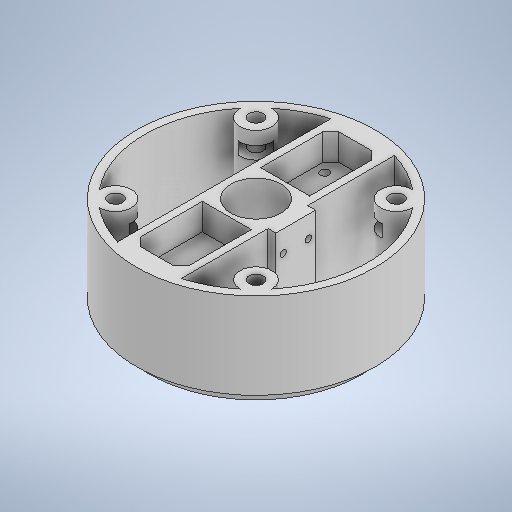
# Autodesk Inventor part: SCARA swivel top
Saved by Autodesk Inventor 2025.2 (Build 292293000, 293)
## iProperties
Created: 2025-01-26
Part Number: SCARA swivel top
Material: Generic
Document SubType Name: Modeling
Designer: caomi
Density: 1 g/cm^3
Appearance: Default
Author: caomi
Autodesk Inventor part; units mm, degrees
ref_plane "YZ Plane" through (0, 0, 0) normal (1, 0, 0) x (0, 1, 0)
ref_plane "XZ Plane" through (0, 0, 0) normal (0, 1, 0) x (-1, 0, 0)
ref_plane "XY Plane" through (0, 0, 0) normal (0, 0, 1) x (1, 0, 0)
sketch "Sketch1" plane through (0, 0, 0) normal (0, 1, 0) x (-1, 0, 0)
  circle A0 centre (0, 0) radius 45
  line L0 (9.25, 37.5) -> (-9.25, 37.5)
  line L1 (-9.25, 37.5) -> (-9.25, 11)
  line L2 (-9.25, 11) -> (9.25, 11)
  line L3 (9.25, 11) -> (9.25, 37.5)
  line L4 (-9.25, -11) -> (9.25, -11)
  line L5 (9.25, -11) -> (9.25, -37.5)
  line L6 (9.25, -37.5) -> (-9.25, -37.5)
  line L7 (-9.25, -37.5) -> (-9.25, -11)
  line L8 (22.2209, 0) -> (-22.2209, 0) construction
  circle A1 centre (0, 0) radius 3
  circle A2 centre (0, 0) radius 9.5
  line L9 (-15.5, -15.5) -> (15.5, -15.5) construction
  line L10 (15.5, -15.5) -> (15.5, 15.5) construction
  line L11 (15.5, 15.5) -> (-15.5, 15.5) construction
  line L12 (-15.5, 15.5) -> (-15.5, -15.5) construction
  line L13 (-15.5, -15.5) -> (15.5, 15.5) construction
  line L14 (15.5, -15.5) -> (-15.5, 15.5) construction
  line L15 (0, 48.862) -> (0, 10.8876) construction
  line L16 (0, -56.5383) -> (0, 11.5383) construction
  circle A3 centre (15.5, 15.5) radius 1.5
  circle A4 centre (15.5, -15.5) radius 1.5
  circle A5 centre (-15.5, -15.5) radius 1.5
  circle A6 centre (-15.5, 15.5) radius 1.5
  line L17 (-5.5, -28.1514) -> (-2.6, -29.8257)
  line L18 (-2.6, -29.8257) -> (-2.6, -33.1743)
  line L19 (-2.6, -33.1743) -> (-5.5, -34.8486)
  line L20 (-5.5, -34.8486) -> (-8.4, -33.1743)
  line L21 (-8.4, -33.1743) -> (-8.4, -29.8257)
  line L22 (-8.4, -29.8257) -> (-5.5, -28.1514)
  line L23 (5.5, -28.1514) -> (8.4, -29.8257)
  line L24 (8.4, -29.8257) -> (8.4, -33.1743)
  line L25 (8.4, -33.1743) -> (5.5, -34.8486)
  line L26 (5.5, -34.8486) -> (2.6, -33.1743)
  line L27 (2.6, -33.1743) -> (2.6, -29.8257)
  line L28 (2.6, -29.8257) -> (5.5, -28.1514)
  line L29 (-5.5, 28.1514) -> (-2.6, 29.8257)
  line L30 (-2.6, 29.8257) -> (-2.6, 33.1743)
  line L31 (-2.6, 33.1743) -> (-5.5, 34.8486)
  line L32 (-5.5, 34.8486) -> (-8.4, 33.1743)
  line L33 (-8.4, 33.1743) -> (-8.4, 29.8257)
  line L34 (-8.4, 29.8257) -> (-5.5, 28.1514)
  line L35 (5.5, 28.1514) -> (8.4, 29.8257)
  line L36 (8.4, 29.8257) -> (8.4, 33.1743)
  line L37 (8.4, 33.1743) -> (5.5, 34.8486)
  line L38 (5.5, 34.8486) -> (2.6, 33.1743)
  line L39 (2.6, 33.1743) -> (2.6, 29.8257)
  line L40 (2.6, 29.8257) -> (5.5, 28.1514)
  circle A7 centre (-5.5, -31.5) radius 1.65
  circle A8 centre (5.5, -31.5) radius 1.65
  circle A9 centre (-5.5, 31.5) radius 1.65
  circle A10 centre (5.5, 31.5) radius 1.65
  point P0 (0, 22.5)
  point P1 (0, -22.5)
  point P2 (0, -22.5)
  point P3 (-2.6, -31.5)
  dimension "d0" = 90
  dimension "d11" = 6
  dimension "d12" = 19
  dimension "d13" = 31
  dimension "d15" = 18.5
  dimension "d16" = 15
  dimension "d17" = 15
  dimension "d18" = 45
  dimension "d19" = 3
  dimension "d23" = 11
  dimension "d25" = 3.3
  dimension "d70" = 9
  dimension "d71" = 26.5
  dimension "d72" = 5.8
  constraints: 82 end point, 18 symmetric about line, 11 centre point, 9 coincident, 6 parallel, 5 midpoint, 4 equal length, 4 equal radius, 4 horizontal, 4 vertical, 3 perpendicular, 2 point on line, 2 vertical alignment, 1 horizontal alignment, 30 other
  measures "d0" diameter of A0
  measures "d11" diameter of A1
  measures "d12" diameter of A2
  measures "d13" distance of L9.end L10.end
  measures "d15" distance of L0.start L0.end
  measures "d16" distance from line of L0 point (0, 22.5)
  measures "d17" distance from line of point (0, -22.5) L6
  measures "d18" distance of point (0, -22.5) point (0, 22.5)
  measures "d19" diameter of A3
  measures "d23" distance of point (-5.5, -31.5) point (5.5, -31.5)
  measures "d25" diameter of A7
  measures "d70" vertical distance of point (0, -22.5) point (-5.5, -31.5)
  measures "d71" distance of L6.end L4.start
  measures "d72" distance from line of point (-2.6, -31.5) L21
extrude "Extrusion1" add sketch "Sketch1" against normal blind 15 contours A0 | L3 L2 L1 L0 | L4 L5 L6 L7 | A2 | A3 | A4 | A5 | A6
extrude "Extrusion4" add sketch "Sketch1" against normal blind 3 contours L17 L18 L19 L20 L21 L22 | L23 L24 L25 L26 L27 L28 | L34 L33 L32 L31 L30 L29 | L40 L39 L38 L37 L36 L35
extrude "Extrusion2" add sketch "Sketch1" along normal blind 20.5 contours A0 | A3 | A4 | A5 | A6
extrude "Extrusion5" add sketch "Sketch1" along normal blind 10.5 contours L3 L2 L1 L0 | L4 L5 L6 L7 | L17 L18 L19 L20 L21 L22 | L23 L24 L25 L26 L27 L28 | L34 L33 L32 L31 L30 L29 | L40 L39 L38 L37 L36 L35
extrude "Extrusion3" cut sketch "Sketch1" along normal through all both and the other way through all contours A3 | A4 | A5 | A6
chamfer "Chamfer1" distance 3 angle 45 4 edges at (-9.25, 15.5, 37.5) (9.25, 15.5, 37.5) (-9.25, 15.5, -37.5) (9.25, 15.5, -37.5)
sketch "Sketch4" plane through (0, -15, 0) normal (0, -1, 0) x (1, 0, 0)
  circle A0 centre (0, 0) radius 11
  dimension "d34" = 22
  constraints: 1 centre point, 1 coincident
  measures "d34" diameter of A0
extrude "Extrusion6" cut sketch "Sketch4" against normal blind 2
sketch "Sketch5" plane through (0, 20.5, 0) normal (0, 1, 0) x (1, 0, 0)
  circle A0 centre (0, 0) radius 3 projected
  circle A1 centre (0, 0) radius 42
  line L0 (-12, -40.2492) -> (-12, 40.2492)
  line L1 (12, 40.2492) -> (12, -40.2492)
  line L2 (0, 51.8199) -> (0, 0) construction
  dimension "d37" = 84
  dimension "d38" = 12
  constraints: 6 end point, 4 point on circle, 3 vertical, 1 centre point, 1 coincident, 1 other
  measures "d37" diameter of A1
  measures "d38" distance between parallel lines of L1 L2
extrude "Extrusion7" cut sketch "Sketch5" against normal blind 30 contours A1 L1 | L0 A1
sketch "Sketch6" plane through (0, 20.5, 0) normal (0, 1, 0) x (1, 0, 0)
  circle A0 centre (-26.5165, 26.5165) radius 6
  line L0 (-26.5165, 26.5165) -> (0, 0) construction
  line L1 (-23.7305, 0) -> (26.8317, 0) construction
  circle A1 centre (-26.5165, -26.5165) radius 6
  line L2 (-26.5165, -26.5165) -> (0, 0) construction
  line L3 (0, 17.9751) -> (0, -18.8342) construction
  circle A2 centre (26.5165, 26.5165) radius 6
  circle A3 centre (26.5165, -26.5165) radius 6
  line L4 (-21.3301, 27.9062) -> (-22.7198, 22.7198)
  line L5 (-22.7198, 22.7198) -> (-27.9062, 21.3301)
  line L6 (-27.9062, 21.3301) -> (-31.7029, 25.1268)
  line L7 (-31.7029, 25.1268) -> (-30.3132, 30.3132)
  line L8 (-30.3132, 30.3132) -> (-25.1268, 31.7029)
  line L9 (-25.1268, 31.7029) -> (-21.3301, 27.9062)
  circle A4 centre (-26.5165, 26.5165) radius 2.65
  line L10 (0, -17.9751) -> (0, 18.8342) construction
  line L11 (-21.3301, -27.9062) -> (-22.7198, -22.7198)
  line L12 (-22.7198, -22.7198) -> (-27.9062, -21.3301)
  line L13 (-27.9062, -21.3301) -> (-31.7029, -25.1268)
  line L14 (-31.7029, -25.1268) -> (-30.3132, -30.3132)
  line L15 (-30.3132, -30.3132) -> (-25.1268, -31.7029)
  line L16 (-25.1268, -31.7029) -> (-21.3301, -27.9062)
  circle A5 centre (-26.5165, -26.5165) radius 2.65
  line L17 (21.3301, 27.9062) -> (22.7198, 22.7198)
  line L18 (22.7198, 22.7198) -> (27.9062, 21.3301)
  line L19 (27.9062, 21.3301) -> (31.7029, 25.1268)
  line L20 (31.7029, 25.1268) -> (30.3132, 30.3132)
  line L21 (30.3132, 30.3132) -> (25.1268, 31.7029)
  line L22 (25.1268, 31.7029) -> (21.3301, 27.9062)
  circle A6 centre (26.5165, 26.5165) radius 2.65
  line L23 (31.7029, -25.1268) -> (30.3132, -30.3132)
  line L24 (27.9062, -21.3301) -> (31.7029, -25.1268)
  line L25 (22.7198, -22.7198) -> (27.9062, -21.3301)
  circle A7 centre (26.5165, -26.5165) radius 2.65
  line L26 (21.3301, -27.9062) -> (22.7198, -22.7198)
  line L27 (25.1268, -31.7029) -> (21.3301, -27.9062)
  line L28 (30.3132, -30.3132) -> (25.1268, -31.7029)
  line L29 (-27.9062, 21.3301) -> (-27.1234, 20.5473)
  line L30 (-21.3301, 27.9062) -> (-20.5473, 27.1234)
  line L31 (-27.9062, -21.3301) -> (-27.1234, -20.5473)
  line L32 (-21.3301, -27.9062) -> (-20.5473, -27.1234)
  line L33 (27.9062, 21.3301) -> (27.1234, 20.5473)
  line L34 (21.3301, 27.9062) -> (20.5473, 27.1234)
  line L35 (27.9062, -21.3301) -> (27.1234, -20.5473)
  line L36 (21.3301, -27.9062) -> (20.5473, -27.1234)
  point P0 (20.5473, 27.1234)
  point P1 (27.1234, 20.5473)
  point P2 (27.1234, -20.5473)
  point P3 (20.5473, -27.1234)
  point P4 (-20.5473, -27.1234)
  dimension "d41" = 37.5
  dimension "d43" = 12
  dimension "d44" = 45
  dimension "d45" = 9.3
  dimension "d46" = 5.3
  constraints: 74 end point, 31 symmetric about line, 8 centre point, 2 coincident, 2 collinear, 2 point on circle, 2 point on line, 1 equal radius, 1 horizontal, 1 vertical, 20 other
  measures "d41" distance of L0.start L0.end
  measures "d43" diameter of A0
  measures "d44" angle of L1 L0
  measures "d45" distance between parallel lines of L8 L5
  measures "d46" diameter of A4
extrude "Extrusion8" add sketch "Sketch6" against normal up to surface (30 mm away)
ref_plane "Work Plane1" through (0, 15.5, 0) normal (0, 1, 0) x (1, 0, 0)
extrude "Extrusion9" cut sketch "Sketch6" against normal blind 4.7 from surface at -5 contours A0 L29 L5 L4 L30 | L4 L5 L6 L7 L8 L9 | A1 L32 L11 L12 L31 | L12 L11 L16 L15 L14 L13 | L34 L17 L18 L33 A2 | L22 L21 L20 L19 L18 L17 | L35 L25 L26 L36 A3 | L24 L23 L28 L27 L26 L25
sketch "Sketch7" plane through (0, -9.5, 0) normal (0, 1, 0) x (1, 0, 0)
  line L0 (-18.5591, 0) -> (20.3221, 0) construction
  line L1 (12, -40.2492) -> (12, 40.2492) projected
  line L2 (12, 7.5) -> (15, 7.5)
  line L3 (15, 7.5) -> (15, -7.5)
  line L4 (15, -7.5) -> (12, -7.5)
  line L5 (12, -7.5) -> (12, 7.5)
  point P0 (0, 0)
  dimension "d61" = 15
  dimension "d62" = 3
  constraints: 10 end point, 2 horizontal, 2 parallel, 2 point on line, 1 perpendicular, 1 other
  measures "d61" distance of L2.end L3.end
  measures "d62" distance between parallel lines of L1 L3
extrude "Extrusion10" add sketch "Sketch7" along normal up to surface (30 mm away)
sketch "Sketch8" plane through (15, -9.5, -7.5) normal (-1, 0, 0) x (0, 0, 1)
  circle A0 centre (12.25, 22) radius 1.2
  circle A1 centre (2.75, 22) radius 1.2
  line L0 (2.75, 22) -> (12.25, 22) construction
  line L1 (7.5, 28.9581) -> (7.5, 20.5932) construction
  line L2 (0, 30) -> (15, 30) projected
  point P0 (7.5, 9.5)
  point P1 (7.5, 30)
  dimension "d56" = 9.5
  dimension "d57" = 2.4
  dimension "d63" = 8
  constraints: 4 end point, 2 centre point, 1 equal radius, 1 horizontal, 1 point on line, 1 vertical, 1 other
  measures "d56" distance of L0.start L0.end
  measures "d57" diameter of A1
  measures "d63" distance between parallel lines of L0 L2
extrude "Extrusion11" cut sketch "Sketch8" along normal blind 5
sketch "Sketch9" plane through (0, -15, 0) normal (0, -1, 0) x (1, 0, 0)
  line L0 (-21.5, -21.5) -> (21.5, -21.5)
  line L1 (21.5, -21.5) -> (21.5, 21.5)
  line L2 (21.5, 21.5) -> (-21.5, 21.5)
  line L3 (-21.5, 21.5) -> (-21.5, -21.5)
  line L4 (-21.5, -21.5) -> (21.5, 21.5) construction
  line L5 (21.5, -21.5) -> (-21.5, 21.5) construction
  circle A0 centre (0, 0) radius 45 projected
  line L6 (8.4, 33.1743) -> (8.4, 29.8257) projected
  line L7 (2.6, 29.8257) -> (2.6, 33.1743) projected
  line L8 (5.5, 28.1514) -> (2.6, 29.8257) projected
  line L9 (8.4, 29.8257) -> (5.5, 28.1514) projected
  line L10 (2.6, 33.1743) -> (5.5, 34.8486) projected
  line L11 (5.5, 34.8486) -> (8.4, 33.1743) projected
  line L12 (-2.6, 33.1743) -> (-2.6, 29.8257) projected
  line L13 (-5.5, 34.8486) -> (-2.6, 33.1743) projected
  line L14 (-8.4, 33.1743) -> (-5.5, 34.8486) projected
  line L15 (-8.4, 29.8257) -> (-8.4, 33.1743) projected
  line L16 (-5.5, 28.1514) -> (-8.4, 29.8257) projected
  line L17 (-2.6, 29.8257) -> (-5.5, 28.1514) projected
  circle A1 centre (-15.5, 15.5) radius 1.5 projected
  circle A2 centre (15.5, 15.5) radius 1.5 projected
  circle A3 centre (15.5, -15.5) radius 1.5 projected
  circle A4 centre (0, 0) radius 11 projected
  circle A5 centre (15.5, 15.5) radius 1.5 projected
  circle A6 centre (-15.5, 15.5) radius 1.5 projected
  circle A7 centre (15.5, -15.5) radius 1.5 projected
  circle A8 centre (-15.5, -15.5) radius 1.5 projected
  circle A9 centre (0, 0) radius 45 projected
  line L18 (8.4, 33.1743) -> (8.4, 29.8257) projected
  line L19 (8.4, 29.8257) -> (5.5, 28.1514) projected
  line L20 (5.5, 28.1514) -> (2.6, 29.8257) projected
  line L21 (2.6, 29.8257) -> (2.6, 33.1743) projected
  line L22 (2.6, 33.1743) -> (5.5, 34.8486) projected
  line L23 (5.5, 34.8486) -> (8.4, 33.1743) projected
  line L24 (-8.4, 29.8257) -> (-8.4, 33.1743) projected
  line L25 (-8.4, 33.1743) -> (-5.5, 34.8486) projected
  line L26 (-5.5, 34.8486) -> (-2.6, 33.1743) projected
  line L27 (-2.6, 33.1743) -> (-2.6, 29.8257) projected
  line L28 (-2.6, 29.8257) -> (-5.5, 28.1514) projected
  line L29 (-5.5, 28.1514) -> (-8.4, 29.8257) projected
  line L30 (2.6, -29.8257) -> (5.5, -28.1514) projected
  line L31 (5.5, -28.1514) -> (8.4, -29.8257) projected
  line L32 (8.4, -29.8257) -> (8.4, -33.1743) projected
  line L33 (8.4, -33.1743) -> (5.5, -34.8486) projected
  line L34 (5.5, -34.8486) -> (2.6, -33.1743) projected
  line L35 (2.6, -33.1743) -> (2.6, -29.8257) projected
  line L36 (-8.4, -29.8257) -> (-5.5, -28.1514) projected
  line L37 (-5.5, -28.1514) -> (-2.6, -29.8257) projected
  line L38 (-2.6, -29.8257) -> (-2.6, -33.1743) projected
  line L39 (-2.6, -33.1743) -> (-5.5, -34.8486) projected
  line L40 (-5.5, -34.8486) -> (-8.4, -33.1743) projected
  line L41 (-8.4, -33.1743) -> (-8.4, -29.8257) projected
  dimension "d64" = 43
  constraints: 12 end point, 2 midpoint, 2 parallel, 2 perpendicular, 1 horizontal
  measures "d64" distance of L1.end L2.end
extrude "Extrusion12" add sketch "Sketch9" along normal blind 2 contours A0
chamfer "Chamfer2" distance 3.5 angle 45 4 edges at (21.5, -16, 21.5) (21.5, -16, -21.5) (-21.5, -16, -21.5) (-21.5, -16, 21.5)
chamfer "Chamfer3" distance 5 angle 45 1 edges at (-45, -17, 0)
body "Solid1"
